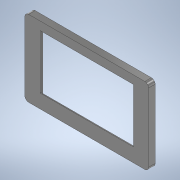
# Autodesk Inventor part: DisplayCover
Saved by Autodesk Inventor 2020 (Build 240168000, 168)
## iProperties
Created: 2021-05-02
Part Number: DisplayCover
Material: ABS Plastic
Document SubType Name: Modeling
Designer: 10300812
Density: 1.06 g/cm^3
Appearance: Anodized - Light Gray
Author: 10300812
Autodesk Inventor part; units mm, degrees
ref_plane "YZ Plane" through (0, 0, 0) normal (1, 0, 0) x (0, 1, 0)
ref_plane "XZ Plane" through (0, 0, 0) normal (0, 1, 0) x (-1, 0, 0)
ref_plane "XY Plane" through (0, 0, 0) normal (0, 0, 1) x (1, 0, 0)
sketch "Sketch1" plane through (0, 0, 0) normal (0, 0, 1) x (1, 0, 0)
  line L0 (-61, 40) -> (61, 40)
  line L1 (65, 36) -> (65, -36)
  line L2 (61, -40) -> (-61, -40)
  line L3 (-65, -36) -> (-65, 36)
  line L4 (-65, 40) -> (65, -40) construction
  line L5 (65, 40) -> (-65, -40) construction
  arc A0 (-61, 40) -> (-65, 36) centre (-61, 36) ccw
  arc A1 (-65, -36) -> (-61, -40) centre (-61, -36) ccw
  arc A2 (61, -40) -> (65, -36) centre (61, -36) ccw
  arc A3 (65, 36) -> (61, 40) centre (61, 36) ccw
  point P0 (0, 0)
  dimension "d0" = 130
  dimension "d1" = 80
  dimension "d2" = 4
  constraints: 12 end point, 8 point on circle, 8 point on line, 8 tangent, 4 centre point, 3 equal radius, 2 midpoint, 2 parallel, 1 horizontal, 1 perpendicular
  measures "d0" distance of L4.end L5.end
  measures "d1" distance of L5.start L4.end
  measures "d2" radius of A0
extrude "Extrusion1" add sketch "Sketch1" along normal blind 6.855
sketch "Sketch2" plane through (0, 0, 6.855) normal (0, 0, 1) x (1, 0, 0)
  line L0 (49.225, 31.315) -> (-48.825, 31.315) projected
  line L1 (-48.825, 31.315) -> (-48.825, -25.535) projected
  line L2 (-48.825, -25.535) -> (49.225, -25.535) projected
  line L3 (49.225, -25.535) -> (49.225, 31.315) projected
  point P0 (0, 0)
extrude "Extrusion2" cut sketch "Sketch2" against normal through all
sketch "Sketch3" plane through (0, 0, 0) normal (0, 0, -1) x (-1, 0, 0)
  line L0 (-52.95, -31.635) -> (-52.95, 31.69) projected
  line L1 (-51.025, 33.615) -> (50.55, 33.615) projected
  line L2 (50.55, 33.615) -> (50.747, 33.615) projected
  line L3 (50.747, 33.615) -> (51.1334, 33.5382) projected
  line L4 (51.1334, 33.5382) -> (51.4974, 33.3874) projected
  line L5 (51.4974, 33.3874) -> (51.8249, 33.1685) projected
  line L6 (51.8249, 33.1685) -> (52.1035, 32.8899) projected
  line L7 (52.1035, 32.8899) -> (52.3224, 32.5624) projected
  line L8 (52.3224, 32.5624) -> (52.4731, 32.1984) projected
  line L9 (52.4731, 32.1984) -> (52.55, 31.812) projected
  line L10 (52.55, 31.812) -> (52.55, 31.615) projected
  line L11 (52.55, 31.615) -> (52.55, -31.635) projected
  line L12 (52.55, -31.635) -> (52.55, -31.827) projected
  line L13 (52.55, -31.827) -> (52.4751, -32.2038) projected
  line L14 (52.4751, -32.2038) -> (52.3281, -32.5587) projected
  line L15 (52.3281, -32.5587) -> (52.1147, -32.878) projected
  line L16 (52.1147, -32.878) -> (51.843, -33.1497) projected
  line L17 (51.843, -33.1497) -> (51.5237, -33.3631) projected
  line L18 (51.5237, -33.3631) -> (51.1688, -33.5101) projected
  line L19 (51.1688, -33.5101) -> (50.7921, -33.585) projected
  line L20 (50.7921, -33.585) -> (50.6, -33.585) projected
  line L21 (50.6, -33.585) -> (-51, -33.585) projected
  line L22 (-52.95, -31.827) -> (-52.95, -31.635) projected
  line L23 (-52.8751, -32.2038) -> (-52.95, -31.827) projected
  line L24 (-52.7281, -32.5587) -> (-52.8751, -32.2038) projected
  line L25 (-52.5147, -32.878) -> (-52.7281, -32.5587) projected
  line L26 (-52.2431, -33.1497) -> (-52.5147, -32.878) projected
  line L27 (-51.9237, -33.3631) -> (-52.2431, -33.1497) projected
  line L28 (-51.5688, -33.5101) -> (-51.9237, -33.3631) projected
  line L29 (-51.1921, -33.585) -> (-51.5688, -33.5101) projected
  line L30 (-51, -33.585) -> (-51.1921, -33.585) projected
  line L31 (-51.2146, 33.615) -> (-51.025, 33.615) projected
  line L32 (-51.5865, 33.541) -> (-51.2146, 33.615) projected
  line L33 (-51.9368, 33.3959) -> (-51.5865, 33.541) projected
  line L34 (-52.2521, 33.1853) -> (-51.9368, 33.3959) projected
  line L35 (-52.5203, 32.9171) -> (-52.2521, 33.1853) projected
  line L36 (-52.7309, 32.6018) -> (-52.5203, 32.9171) projected
  line L37 (-52.876, 32.2515) -> (-52.7309, 32.6018) projected
  line L38 (-52.95, 31.8796) -> (-52.876, 32.2515) projected
  line L39 (-52.95, 31.69) -> (-52.95, 31.8796) projected
  line L40 (50.55, 33.865) -> (-51.025, 33.865)
  line L41 (-51.025, 33.865) -> (-51.2392, 33.865)
  line L42 (-51.2392, 33.865) -> (-51.6594, 33.7814)
  line L43 (-51.6594, 33.7814) -> (-52.0553, 33.6175)
  line L44 (-52.0553, 33.6175) -> (-52.4115, 33.3794)
  line L45 (-52.4115, 33.3794) -> (-52.7144, 33.0765)
  line L46 (-52.7144, 33.0765) -> (-52.9525, 32.7203)
  line L47 (-52.9525, 32.7203) -> (-53.1164, 32.3244)
  line L48 (-53.1164, 32.3244) -> (-53.2, 31.9042)
  line L49 (-53.2, 31.9042) -> (-53.2, 31.69)
  line L50 (-53.2, 31.69) -> (-53.2, -31.635)
  line L51 (-53.2, -31.635) -> (-53.2, -31.8517)
  line L52 (-53.2, -31.8517) -> (-53.1155, -32.2767)
  line L53 (-53.1155, -32.2767) -> (-52.9496, -32.6771)
  line L54 (-52.9496, -32.6771) -> (-52.7089, -33.0374)
  line L55 (-52.7089, -33.0374) -> (-52.4024, -33.3438)
  line L56 (-52.4024, -33.3438) -> (-52.0421, -33.5846)
  line L57 (-52.0421, -33.5846) -> (-51.6417, -33.7504)
  line L58 (-51.6417, -33.7504) -> (-51.2167, -33.835)
  line L59 (-51.2167, -33.835) -> (-51, -33.835)
  line L60 (-51, -33.835) -> (50.6, -33.835)
  line L61 (50.6, -33.835) -> (50.8167, -33.835)
  line L62 (50.8167, -33.835) -> (51.2417, -33.7504)
  line L63 (51.2417, -33.7504) -> (51.6421, -33.5846)
  line L64 (51.6421, -33.5846) -> (52.0024, -33.3438)
  line L65 (52.0024, -33.3438) -> (52.3088, -33.0374)
  line L66 (52.3088, -33.0374) -> (52.5496, -32.6771)
  line L67 (52.5496, -32.6771) -> (52.7155, -32.2767)
  line L68 (52.7155, -32.2767) -> (52.8, -31.8517)
  line L69 (52.8, -31.8517) -> (52.8, -31.635)
  line L70 (52.8, -31.635) -> (52.8, 31.615)
  line L71 (52.8, 31.615) -> (52.8, 31.8366)
  line L72 (52.8, 31.8366) -> (52.7135, 32.2713)
  line L73 (52.7135, 32.2713) -> (52.5439, 32.6808)
  line L74 (52.5439, 32.6808) -> (52.2977, 33.0493)
  line L75 (52.2977, 33.0493) -> (51.9843, 33.3627)
  line L76 (51.9843, 33.3627) -> (51.6158, 33.6089)
  line L77 (51.6158, 33.6089) -> (51.2063, 33.7785)
  line L78 (51.2063, 33.7785) -> (50.7716, 33.865)
  line L79 (50.7716, 33.865) -> (50.55, 33.865)
  point P0 (0, 0)
  dimension "d7" = 0.25
  constraints: 80 end point, 39 other
  measures "d7" distance between parallel lines of L1 L40
extrude "Extrusion3" cut sketch "Sketch3" against normal blind 5.855 contours L0 L39 L38 L37 L36 L35 L34 L33 L32 L31 L1 L2 L3 L4 L5 L6 L7 L8 L9 L10 L11 L12 L13 L14 L15 L16 L17 L18 L19 L20 L21 L30 L29 L28 L27 L26 L25 L24 L23 L22 | L79 L78 L77 L76 L75 L74 L73 L72 L71 L70 L69 L68 L67 L66 L65 L64 L63 L62 L61 L60 L59 L58 L57 L56 L55 L54 L53 L52 L51 L50 L49 L48 L47 L46 L45 L44 L43 L42 L41 L40
sketch "Sketch4" plane through (0, 0, 0) normal (0, 0, -1) x (-1, 0, 0)
  line L0 (-58.1378, 13.8535) -> (-62.7167, 13.8535)
  line L1 (-62.7167, 13.8535) -> (-62.7167, 7.4621)
  line L2 (-62.7167, 7.4621) -> (-58.1378, 7.4621)
  line L3 (-58.1378, 7.4621) -> (-58.1378, 13.8535)
  line L4 (-58.1378, 13.8535) -> (-62.7167, 7.4621) construction
  line L5 (-62.7167, 13.8535) -> (-58.1378, 7.4621) construction
  line L6 (-57.8993, -7.1808) -> (-62.9552, -7.1808)
  line L7 (-62.9552, -7.1808) -> (-62.9552, -13.763)
  line L8 (-62.9552, -13.763) -> (-57.8993, -13.763)
  line L9 (-57.8993, -13.763) -> (-57.8993, -7.1808)
  line L10 (-57.8993, -7.1808) -> (-62.9552, -13.763) construction
  line L11 (-62.9552, -7.1808) -> (-57.8993, -13.763) construction
  point P0 (0, 0)
  point P1 (-60.4272, 10.6578)
  point P2 (-60.4272, -10.4719)
  constraints: 24 end point, 4 midpoint, 4 parallel, 2 horizontal, 2 perpendicular
extrude "Extrusion4" cut sketch "Sketch4" against normal blind 3
sketch "Sketch5" plane through (0, 0, 0) normal (0, 0, -1) x (-1, 0, 0)
  circle A0 centre (61, 36) radius 1.625 projected
  circle A1 centre (61, -36) radius 1.625 projected
  circle A2 centre (-61, -36) radius 1.625 projected
  circle A3 centre (-61, 36) radius 1.625 projected
  point P0 (0, 0)
  constraints: 4 coincident
hole "Hole1" at (61, 36, 0) at (61, -36, 0) at (-61, 36, 0) at (-61, -36, 0) direction (0, 0, 1) diameter 2.459 depth 5.5 thread size "M3x0.5" class "6H" standard "ANSI Metric M Profile"
body "Solid1"
